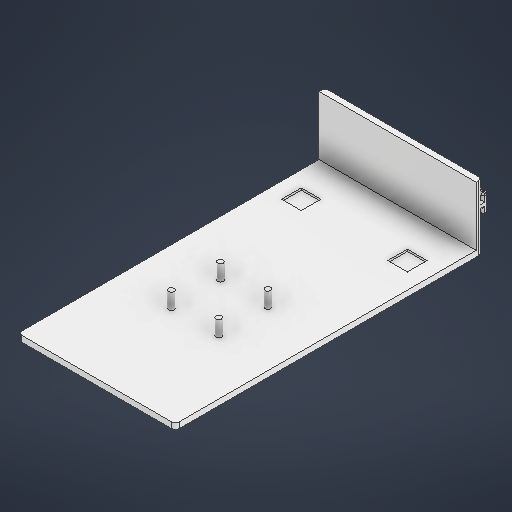
# Autodesk Inventor part: module_command
Saved by Autodesk Inventor 2025.4 (Build 294407000, 407)
## iProperties
Created: 2025-09-05
Part Number: module_command
Material: PC/ABS Plastic
Document SubType Name: Modeling
Designer: sam
Density: 1.1 g/cm^3
Appearance: Smooth - White
Author: sam
Autodesk Inventor part; units mm, degrees
ref_plane "YZ Plane" through (0, 0, 0) normal (1, 0, 0) x (0, 1, 0)
ref_plane "XZ Plane" through (0, 0, 0) normal (0, 1, 0) x (-1, 0, 0)
ref_plane "XY Plane" through (0, 0, 0) normal (0, 0, 1) x (1, 0, 0)
sketch "Sketch1" plane through (0, 0, 0) normal (0, 1, 0) x (-1, 0, 0)
  line L0 (-40, -78) -> (40, -78)
  line L1 (40, -78) -> (40, 78)
  line L2 (40, 78) -> (-40, 78)
  line L3 (-40, 78) -> (-40, -78)
  line L4 (-40, -78) -> (40, 78) construction
  line L5 (40, -78) -> (-40, 78) construction
  point P0 (0, 0)
  dimension "d0" = 80
  dimension "d1" = 156
  constraints: 12 end point, 2 midpoint, 2 parallel, 1 horizontal, 1 perpendicular
  measures "d0" distance of L2.end L1.end
  measures "d1" distance of L1.end L0.end
extrude "Extrusion1" add sketch "Sketch1" along normal blind 3
sketch "Sketch2" plane through (0, 3, 0) normal (0, 1, 0) x (1, 0, 0)
  line L0 (-40, 78) -> (-40, -78) projected
  line L1 (-40, -78) -> (40, -78) projected
  line L2 (40, -78) -> (40, 78) projected
  line L3 (40, 78) -> (-40, 78) projected
  line L4 (40, 78) -> (-40, 78)
  line L5 (-40, 78) -> (-40, -78)
  line L6 (-40, -78) -> (40, -78)
  line L7 (40, -78) -> (40, 78)
  line L8 (40, 78) -> (-40, -78) construction
  line L9 (-40, 78) -> (40, -78) construction
  line L10 (37, 75) -> (-37, 75)
  line L11 (-37, 75) -> (-37, -75)
  line L12 (-37, -75) -> (37, -75)
  line L13 (37, -75) -> (37, 75)
  line L14 (37, 75) -> (-37, -75) construction
  line L15 (-37, 75) -> (37, -75) construction
  point P0 (0, 0)
  dimension "d4" = 0
  dimension "d5" = 0
  dimension "d6" = 3
  dimension "d7" = 3
  constraints: 24 end point, 4 midpoint, 4 parallel, 2 horizontal, 2 perpendicular
  measures "d4" distance between parallel lines of L0 L5
  measures "d5" distance between parallel lines of L1 L6
  measures "d6" distance between parallel lines of L5 L11
  measures "d7" distance between parallel lines of L6 L12
extrude "Extrusion2" add sketch "Sketch2" along normal blind 30
fillet "Fillet1" radius 2 4 edges at (40, 16.5, 78) (40, 16.5, -78) (-40, 16.5, 78) (-40, 16.5, -78)
sketch "Sketch13" plane through (23.2, 5, -78) normal (0, 0, -1) x (-1, 0, 0)
  line L0 (-13.8, 18) -> (60.2, 18)
  line L1 (60.2, 18) -> (60.2, 8.4)
  line L2 (60.2, 8.4) -> (-13.8, 8.4)
  line L3 (-13.8, 8.4) -> (-13.8, 18)
  line L4 (63.2, -5) -> (63.2, 28) projected
  line L5 (-16.8, 28) -> (-16.8, -5) projected
  line L6 (-14.8, -5) -> (61.2, -5) projected
  point P0 (23.2, -5)
  point P1 (51.4, 0)
  point P2 (-5, 0)
  point P3 (-16.8, -5)
  point P4 (63.2, 11.5)
  point P5 (60.2, 13.2)
  dimension "d131" = 9.6
  dimension "d146" = 3
  dimension "d147" = 3
  dimension "d156" = 23
  constraints: 8 end point, 2 parallel, 1 horizontal, 1 midpoint, 1 perpendicular, 3 other
  measures "d131" distance of L0.end L1.end
  measures "d156" distance between parallel lines of L0 L6
extrude "Extrusion13" add sketch "Sketch13" along normal blind 6
sketch "Sketch14" plane through (-37, 13.4, -78) normal (-1, 0, 0) x (0, 0, 1)
  line L0 (0, 9.6) -> (0, 0) projected
  line L1 (0, 9.6) -> (-6, 9.6) projected
  line L2 (-6, 0) -> (-6, 9.6) projected
  line L3 (0, 0) -> (-6, 0) projected
  line L4 (0, 9.6) -> (-3.4, 9.6)
  line L5 (-3.4, 9.6) -> (-3.4, 6.6)
  line L6 (-3.4, 6.6) -> (0, 6.6)
  line L7 (0, 6.6) -> (0, 9.6)
  line L8 (0, 0) -> (-3.4, 0)
  line L9 (-3.4, 0) -> (-3.4, 3)
  line L10 (-3.4, 3) -> (0, 3)
  line L11 (0, 3) -> (0, 0)
  point P0 (78, -13.4)
  point P1 (0, 6.6)
  dimension "d137" = 3.4
  dimension "d138" = 3
  dimension "d139" = 3.4
  dimension "d140" = 3
  constraints: 16 end point, 4 parallel, 2 horizontal, 2 perpendicular
  measures "d137" distance of L6.end L5.end
  measures "d138" distance of L5.end L4.end
  measures "d139" distance of L9.end L10.end
  measures "d140" distance of L8.end L9.end
extrude "Extrusion14" cut sketch "Sketch14" against normal up to surface (74 mm away) contours L0 L6 L5 L1 | L0 L3 L9 L10
fillet "Fillet5" radius 1 18 edges at (0, 23, -84) (0, 23, -81.4) (0, 13.4, -84) (0, 13.4, -81.4) (-37, 16.4, -79.7) (-37, 20, -79.7) (37, 16.4, -79.7) (37, 20, -79.7) (-37, 18.2, -84) (-37, 21.5, -81.4) (-37, 14.9, -81.4) (-37, 23, -82.7) (-37, 13.4, -82.7) (37, 23, -82.7) (37, 13.4, -82.7) (37, 14.9, -81.4) (37, 18.2, -84) (37, 21.5, -81.4)
sketch "Sketch16" plane through (0, 33, 0) normal (0, 1, 0) x (1, 0, 0)
  arc A0 (-38, 78) -> (-40, 76) centre (-38, 76) ccw projected
  line L0 (-40, 76) -> (-40, -76) projected
  arc A1 (-40, -76) -> (-38, -78) centre (-38, -76) ccw projected
  line L1 (-38, -78) -> (38, -78) projected
  arc A2 (38, -78) -> (40, -76) centre (38, -76) ccw projected
  line L2 (40, -76) -> (40, 76) projected
  arc A3 (40, 76) -> (38, 78) centre (38, 76) ccw projected
  line L3 (38, 78) -> (-38, 78) projected
  line L4 (37, 75) -> (37, -75) projected
  line L5 (37, -75) -> (-37, -75) projected
  line L6 (-37, -75) -> (-37, 75) projected
  line L7 (-37, 75) -> (37, 75) projected
  line L8 (-37, 75) -> (-40, 75)
  line L9 (37, 75) -> (40, 75)
  circle A4 centre (38, 76) radius 2
  circle A5 centre (-38, 76) radius 2
  point P0 (0, 0)
  point P1 (-39.7321, 75)
  point P2 (40, 76)
  point P3 (39.7321, 75)
  dimension "d180" = 4
  dimension "d181" = 4
  constraints: 4 end point, 3 point on line, 2 centre point, 2 coincident, 1 perpendicular
  measures "d180" diameter of A4
  measures "d181" diameter of A5
extrude "Extrusion16" cut sketch "Sketch16" against normal blind 30 contours L8 A5 L6 L5 L4 A4 L9 L2 A2 L1 A1 L0 | L8 L6 A5 | A4 L4 L9
sketch "Sketch18" plane through (0, 3, 0) normal (0, 1, 0) x (1, 0, 0)
  line L0 (40, 75) -> (-40, 75) projected
  line L1 (38, -78) -> (-38, -78) projected
  line L2 (40, 75) -> (40, -76) projected
  line L3 (32, 58) -> (22, 58)
  line L4 (22, 58) -> (22, 48)
  line L5 (22, 48) -> (32, 48)
  line L6 (32, 48) -> (32, 58)
  line L7 (-22, 48) -> (-32, 48)
  line L8 (-32, 48) -> (-32, 58)
  line L9 (-32, 58) -> (-22, 58)
  line L10 (-22, 58) -> (-22, 48)
  line L11 (38, 78) -> (-38, 78) projected
  line L12 (-40, -76) -> (-40, 75) projected
  arc A0 (-40, -76) -> (-38, -78) centre (-38, -76) ccw projected
  arc A1 (38, -78) -> (40, -76) centre (38, -76) ccw projected
  dimension "d182" = 10
  dimension "d183" = 10
  dimension "d184" = 8
  dimension "d185" = 10
  dimension "d186" = 10
  dimension "d188" = 20
  dimension "d189" = 20
  constraints: 16 end point, 4 parallel, 2 horizontal, 2 perpendicular
  measures "d182" distance of L5.end L4.end
  measures "d183" distance between parallel lines of L3 L5
  measures "d184" distance between parallel lines of L2 L6
  measures "d185" distance of L8.end L9.end
  measures "d186" distance of L7.end L8.end
  measures "d188" distance between parallel lines of L11 L9
  measures "d189" distance between parallel lines of L11 L3
extrude "Extrusion18" cut sketch "Sketch18" against normal blind 1 contours L6 L5 L4 L3 | L7 L8 L9 L10
sketch "Sketch19" plane through (0, 3, 0) normal (0, 1, 0) x (1, 0, 0)
  line L0 (40, 75) -> (40, -76) projected
  line L1 (38, -78) -> (-38, -78) projected
  line L2 (-40, -76) -> (-40, 76) projected
  circle A0 centre (-12.05, -3) radius 1.45
  circle A1 centre (-12.05, -28) radius 1.45
  circle A2 centre (12.05, -3) radius 1.45
  circle A3 centre (12.05, -28) radius 1.45
  line L3 (-5, -54) -> (5, -54) projected
  line L4 (32, 58) -> (32, 48) projected
  line L5 (-32, 48) -> (-32, 58) projected
  point P0 (40, 76)
  point P1 (0, -54)
  point P2 (0, -54)
  point P3 (32, 53)
  point P4 (-32, 53)
  dimension "d215" = 2.9
  dimension "d216" = 2.9
  dimension "d217" = 2.9
  dimension "d218" = 2.9
  dimension "d219" = 25
  dimension "d220" = 25
  dimension "d221" = 24.1
  dimension "d222" = 12.05
  dimension "d223" = 12.05
  dimension "d224" = 56
  dimension "d225" = 56
  constraints: 4 centre point, 4 midpoint
  measures "d215" diameter of A0
  measures "d216" diameter of A1
  measures "d217" diameter of A2
  measures "d218" diameter of A3
  measures "d219" distance of A2.centre A3.centre
  measures "d220" distance of A0.centre A1.centre
  measures "d221" distance of A2.centre A0.centre
  measures "d222" horizontal distance of point (0, -54) A3.centre
  measures "d223" horizontal distance of point (0, -54) A1.centre
  measures "d224" vertical distance of point (32, 53) A2.centre
  measures "d225" vertical distance of point (-32, 53) A0.centre
extrude "Extrusion19" add sketch "Sketch19" along normal blind 8
body "Solid1"
